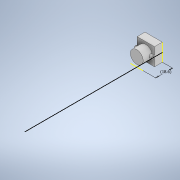
# Autodesk Inventor part: HDzero micro dummy
Saved by Autodesk Inventor 2020 (Build 240168000, 168)
## iProperties
Created: 2022-05-06
Part Number: HDzero micro dummy
Material: Generic
Document SubType Name: Modeling
Designer: Steven
Density: 1 g/cm^3
Appearance: Default
Author: Steven
Autodesk Inventor part; units mm, degrees
ref_plane "YZ Plane" through (0, 0, 0) normal (1, 0, 0) x (0, 1, 0)
ref_plane "XZ Plane" through (0, 0, 0) normal (0, 1, 0) x (-1, 0, 0)
ref_plane "XY Plane" through (0, 0, 0) normal (0, 0, 1) x (1, 0, 0)
sketch "Sketch1" plane through (0, 0, 0) normal (0, 0, 1) x (1, 0, 0)
  line L0 (0, 0) -> (19.1, 0)
  line L1 (19.1, 0) -> (19.1, 19.1)
  line L2 (19.1, 19.1) -> (0, 19.1)
  line L3 (0, 19.1) -> (0, 0)
  dimension "d0" = 19.1
  dimension "d1" = 19.1
  constraints: 8 end point, 2 parallel, 1 horizontal, 1 perpendicular
  measures "d0" distance of L2.end L1.end
  measures "d1" distance of L1.end L0.end
extrude "Extrusion1" add sketch "Sketch1" along normal blind 8.67
sketch "Sketch2" plane through (19.1, 0, 0) normal (1, 0, 0) x (0, 0, -1)
  line L0 (0, 0) -> (0, 19.1) projected
  line L1 (0, 19.1) -> (-8.67, 19.1) projected
  line L2 (-8.67, 0) -> (-8.67, 19.1) projected
  line L3 (0, 0) -> (-8.67, 0) projected
  line L4 (0, 0) -> (0, 19.1) construction
  line L5 (0, 9.55) -> (-11, 9.55) construction
  line L6 (-11, 9.55) -> (-11, 16.3311) construction
  circle A0 centre (-10, 9.55) radius 1
  circle A1 centre (-10, 9.55) radius 2
  point P0 (-8.67, 11.0437)
  point P1 (-8.67, 8.0563)
  dimension "d4" = 11
  dimension "d5" = 2
  dimension "d6" = 4
  constraints: 4 end point, 2 centre point, 1 coincident, 1 horizontal, 1 midpoint, 1 point on line, 1 tangent, 1 vertical
  measures "d4" distance of L5.start L5.end
  measures "d5" diameter of A0
  measures "d6" diameter of A1
extrude "Extrusion2" add sketch "Sketch2" against normal up to surface (19.1 mm away) contours A1 L2 picked at (-8.78, 9.55)
sketch "Sketch3" plane through (0, 0, 8.67) normal (0, 0, 1) x (1, 0, 0)
  line L0 (0, 11.0437) -> (19.1, 11.0437) projected
  line L1 (19.1, 11.0437) -> (19.1, 19.1) projected
  line L2 (19.1, 19.1) -> (0, 19.1) projected
  line L3 (0, 19.1) -> (0, 11.0437) projected
  line L4 (19.1, 8.0563) -> (0, 8.0563) projected
  line L5 (0, 8.0563) -> (0, 0) projected
  line L6 (0, 0) -> (19.1, 0) projected
  line L7 (19.1, 0) -> (19.1, 8.0563) projected
  line L8 (19.1, 19.1) -> (0, 19.1) construction
  line L9 (9.55, 19.1) -> (9.55, 0) construction
  circle A0 centre (9.55, 9.55) radius 7
  dimension "d9" = 14
  constraints: 3 midpoint, 2 end point, 1 centre point
  measures "d9" diameter of A0
extrude "Extrusion3" add sketch "Sketch3" along normal blind 9.93 contours A0 L0 | L0 A0 L4 | L4 A0
sketch "Sketch4" plane through (0, 0, 0) normal (0, -1, 0) x (1, 0, 0)
  line L0 (0, 0) -> (19.1, 0) projected
  line L1 (16.55, 18.6) -> (2.55, 18.6) projected
  dimension "d12" = 18.6
  measures "d12" distance between parallel lines of L0 L1
sketch "Sketch5" plane through (19.1, 0, 0) normal (1, 0, 0) x (0, 0, -1)
  line L0 (0, 0) -> (0, 19.1) projected
  line L1 (0, 9.55) -> (-151.3307, 9.55)
  constraints: 2 end point, 1 horizontal, 1 midpoint
body "Solid1"
